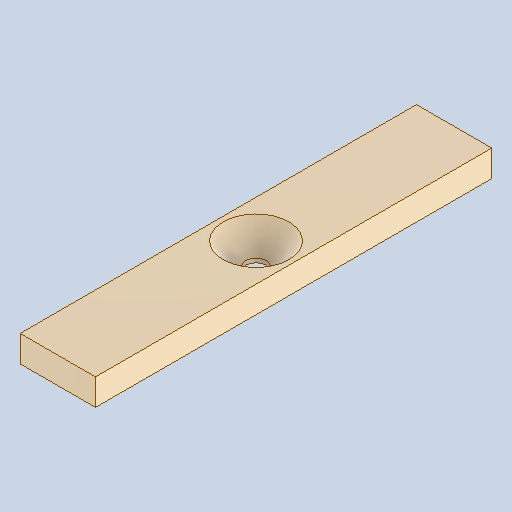
# Autodesk Inventor part: LagerHH
Saved by Autodesk Inventor 2025 (Build 290162010, 162A)
## iProperties
Created: 2024-11-12
Part Number: LagerHH
Material: Polyethylen, hohe Dichte, Gleitfläche
Document SubType Name: Modeling
Designer: Admin
Density: 0.952 g/cm^3
Appearance: Glatt - Eierschale(1)
Author: Admin
Autodesk Inventor part; units mm, degrees
ref_plane "YZ Plane" through (0, 0, 0) normal (1, 0, 0) x (0, 1, 0)
ref_plane "XZ Plane" through (0, 0, 0) normal (0, 1, 0) x (-1, 0, 0)
ref_plane "XY Plane" through (0, 0, 0) normal (0, 0, 1) x (1, 0, 0)
sketch "Skizze1" plane through (0, 0, 0) normal (0, 0, 1) x (1, 0, 0)
  circle A0 centre (2.85, 15) radius 0.7835 projected
  line L0 (0, 0) -> (5.7, 0) projected
  line L1 (5.7, 0) -> (5.7, 30) projected
  line L2 (0, 30) -> (5.7, 30) projected
  line L3 (0, 0) -> (0, 30) projected
extrude "Extrusion1" add sketch "Skizze1" along normal blind 2
chamfer "Fasen1" distance 1.7 angle 45 1 edges at (2.0665, 15, 2)
